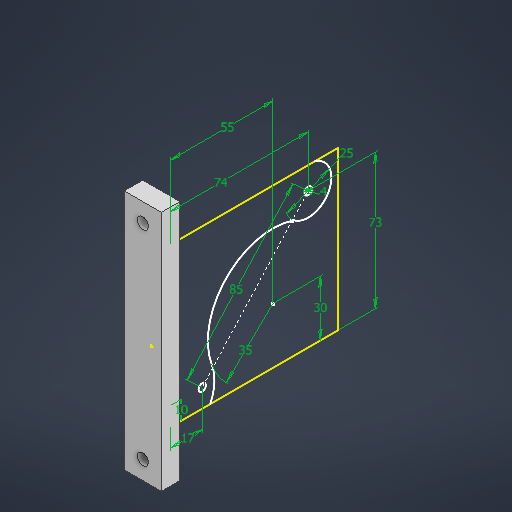
# Autodesk Inventor part: Caliper Bracket Mount
Saved by Autodesk Inventor 2026.1 (Build 301233000, 233)
## iProperties
Created: 2026-06-24
Part Number: Caliper Bracket Mount
Material: Generic
Document SubType Name: Modeling
Designer: share
Density: 1 g/cm^3
Appearance: Default
Author: share
Autodesk Inventor part; units mm, degrees
ref_plane "YZ Plane" through (0, 0, 0) normal (1, 0, 0) x (0, 1, 0)
ref_plane "XZ Plane" through (0, 0, 0) normal (0, 1, 0) x (-1, 0, 0)
ref_plane "XY Plane" through (0, 0, 0) normal (0, 0, 1) x (1, 0, 0)
sketch "Sketch1" plane through (0, 0, 0) normal (0, 0, 1) x (1, 0, 0)
  line L0 (-10, -65) -> (10, -65)
  line L1 (10, -65) -> (10, 65)
  line L2 (10, 65) -> (-10, 65)
  line L3 (-10, 65) -> (-10, -65)
  line L4 (-10, -65) -> (10, 65) construction
  line L5 (10, -65) -> (-10, 65) construction
  line L6 (0, 65) -> (0, -65) construction
  circle A0 centre (0, 55) radius 3
  circle A1 centre (0, -55) radius 3
  line L7 (10, 0) -> (-10, 0) construction
  point P0 (0, 0)
  dimension "d0" = 130
  dimension "d1" = 20
  dimension "d2" = 110
  dimension "d3" = 6
  constraints: 16 end point, 6 midpoint, 2 centre point, 2 parallel, 2 point on line, 1 horizontal, 1 perpendicular, 1 other
  measures "d0" distance between parallel lines of L0 L2
  measures "d1" distance between parallel lines of L1 L3
  measures "d2" distance of A1.centre A0.centre
  measures "d3" diameter of A0
extrude "Base" add sketch "Sketch1" against normal blind 10
sketch "Sketch6" plane through (0, 0, 0) normal (1, 0, 0) x (0, 1, 0)
  line L0 (65, -10) -> (-65, -10) projected
  line L1 (42.5, -10) -> (-42.5, -10)
  line L2 (-42.5, -10) -> (-42.5, -100)
  line L3 (-42.5, -100) -> (42.5, -100)
  line L4 (42.5, -100) -> (42.5, -10)
  line L5 (0, 0) -> (0, -10) construction
  point P0 (-42.5, -10)
  dimension "d69" = 85
  dimension "d70" = 90
  constraints: 10 end point, 2 parallel, 2 perpendicular, 1 horizontal, 1 midpoint, 1 point on line, 1 other
  measures "d69" distance between parallel lines of L2 L4
  measures "d70" distance between parallel lines of L3 L0
extrude "Bracket Mount" add sketch "Sketch6" along normal mid plane 10
sketch "Sketch7" plane through (5, 0, 0) normal (1, 0, 0) x (0, 0, -1)
  line L0 (100, 42.5) -> (10, 42.5) projected
  line L1 (10, -42.5) -> (10, 42.5) projected
  line L2 (10, -42.5) -> (100, -42.5) projected
  line L3 (100, -42.5) -> (100, 42.5) projected
  circle A0 centre (84, 30.5) radius 2
  circle A1 centre (27, -32.5555) radius 2
  line L4 (84, 30.5) -> (27, -32.5555) construction
  arc A2 (76.3633, 20.604) -> (32.1072, -24.461) centre (65, -12.5) ccw
  arc A3 (31.2921, -42.5) -> (32.1072, -24.461) centre (10, -32.5) ccw
  arc A4 (75.6176, 21.2271) -> (87.5, 42.5) centre (84, 30.5) ccw
  point P0 (0, 0)
  point P1 (75.3526, 20.9339)
  dimension "d73" = 85
  dimension "d74" = 4
  dimension "d75" = 74
  dimension "d76" = 73
  dimension "d77" = 17
  dimension "d78" = 30
  dimension "d79" = 55
  dimension "d83" = 35
  dimension "d91" = 10
  dimension "d98" = 25
  constraints: 8 point on circle, 5 centre point, 5 point on line, 2 end point, 1 coincident, 1 equal radius, 1 tangent
  measures "d73" distance of L4.start L4.end
  measures "d74" diameter of A0
  measures "d75" distance from line of L1 L4.start
  measures "d76" distance from line of L4.start L2
  measures "d77" distance from line of L1 L4.end
  measures "d78" distance from line of L2 A2.centre
  measures "d79" distance from line of A2.centre L1
  measures "d83" radius of A2
  measures "d91" distance from line of L2 A3.centre
  measures "d98" diameter of A4
extrude "Cut" cut sketch "Sketch7" against normal through all contours L3 L2 A3 A2 A4 L0 | A4 A2 A3 L2 L1 L0 | A0 | A1
extrude "Mount Holes" cut sketch "Sketch7" against normal through all contours A0 | A1
equation "\"d0\" = Main_Body_Height"
equation "\"d1\" = Main_Body_Width"
equation "\"d2\" = Upright_Hole_Spacing"
equation "\"d69\" = Caliper_Bracket_Mount_Height"
equation "\"d70\" = Caliper_Bracket_Mount_Width"
equation "\"d71\" = Caliper_Bracket_Mount_Thickness"
equation "\"Base_Thickness\" = 4"
equation "\"Main_Body_Height\" = 130"
equation "\"Main_Body_Width\" = 20"
equation "\"Upright_Hole_Spacing\" = 110"
equation "\"Caliper_Bracket_Mount_Thickness\" = 10"
equation "\"Caliper_Bracket_Mount_Width\" = 90"
equation "\"Caliper_Bracket_Mount_Height\" = 85"
body "Solid1"
